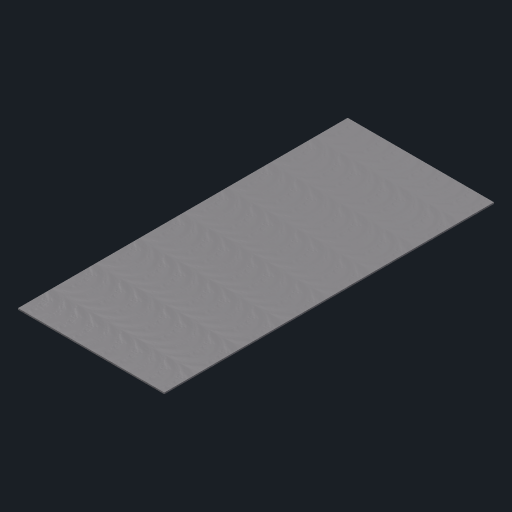
# Autodesk Inventor part: COMPUERTA_ALUMINIO
Saved by Autodesk Inventor 2024.3 (Build 283343000, 343)
## iProperties
Created: 2024-07-04
Part Number: COMPUERTA_ALUMINIO
Material: Steel, Mild, Welded
Document SubType Name: Modeling
Designer: Niler
Density: 7.85 g/cm^3
Appearance: Weld - Steel Mild
Author: Niler
Autodesk Inventor part; units mm, degrees
ref_plane "YZ Plane" through (0, 0, 0) normal (1, 0, 0) x (0, 1, 0)
ref_plane "XZ Plane" through (0, 0, 0) normal (0, 1, 0) x (-1, 0, 0)
ref_plane "XY Plane" through (0, 0, 0) normal (0, 0, 1) x (1, 0, 0)
sketch "Sketch1" plane through (0, 0, 0) normal (0, 1, 0) x (-1, 0, 0)
  line L0 (0, 110) -> (0, -110) construction
  line L1 (-59, 110) -> (-59, -110)
  line L2 (59, -110) -> (59, 110)
  arc A0 (59, 110) -> (-59, 110) centre (0, 110) ccw
  arc A1 (-59, -110) -> (59, -110) centre (0, -110) ccw
  line L3 (-75, 169) -> (75, 169)
  line L4 (75, 169) -> (75, -169)
  line L5 (75, -169) -> (-75, -169)
  line L6 (-75, -169) -> (-75, 169)
  line L7 (-75, 169) -> (75, -169) construction
  line L8 (75, 169) -> (-75, -169) construction
  point P0 (0, 0)
  point P1 (0, -169)
  point P2 (0, 169)
  dimension "d0" = 118
  dimension "d1" = 220
  dimension "d4" = 150
  constraints: 20 end point, 5 point on circle, 4 midpoint, 4 tangent, 3 parallel, 2 centre point, 1 horizontal, 1 perpendicular, 1 vertical
  measures "d0" distance between parallel lines of L1 L2
  measures "d1" distance of L0.start L0.end
  measures "d4" distance of L4.end L5.end
extrude "Extrusion1" add sketch "Sketch1" along normal blind 1.5
body "Solid1"
